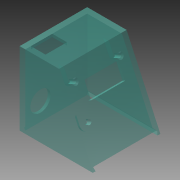
# Autodesk Inventor part: Caja temporizador
Saved by Autodesk Inventor 2014 (Build 180170000, 170)
## iProperties
Created: 2017-07-04
Part Number: Caja temporizador
Material: Generic
Document SubType Name: Modeling
Designer: resaj
Density: 1 g/cm^3
Appearance: Indoor Pool
Author: resaj
Autodesk Inventor part; units mm, degrees
ref_plane "YZ Plane" through (0, 0, 0) normal (1, 0, 0) x (0, 1, 0)
ref_plane "XZ Plane" through (0, 0, 0) normal (0, 1, 0) x (-1, 0, 0)
sketch "Sketch1" plane through (0, 0, 0) normal (0, 0, 1) x (1, 0, 0)
  line L0 (0, 0) -> (0, 65)
  line L1 (0, 65) -> (35, 65)
  line L2 (35, 65) -> (65, 0)
  line L3 (65, 0) -> (0, 0)
  line L4 (35, 65) -> (19.5647, 57.876) construction
  line L5 (19.5647, 57.876) -> (40.0985, 13.386) construction
  line L6 (40.0985, 13.386) -> (55.5339, 20.51) construction
  line L7 (5, 65) -> (5, 39) construction
  line L8 (5, 39) -> (17.8, 39) construction
  line L9 (17.8, 39) -> (17.8, 65) construction
  line L10 (0, 23.6) -> (40, 23.6) construction
  line L11 (40, 23.6) -> (40, 6) construction
  line L12 (40, 6) -> (0, 6) construction
  line L13 (0, 26.5) -> (11, 26.5) construction
  line L14 (11, 26.5) -> (11, 23.6) construction
  line L15 (11, 6) -> (11, 3.1) construction
  line L16 (11, 3.1) -> (0, 3.1) construction
  dimension "d27" = 17
  dimension "d28" = 12.8
  dimension "d29" = 5
  dimension "d31" = 40
  dimension "d32" = 17.6
  dimension "d33" = 26
  dimension "d34" = 35
  dimension "d35" = 65
  dimension "d36" = 23.4
  dimension "d37" = 11
  dimension "d38" = 49
  dimension "d39" = 65
  dimension "d40" = 6
  constraints: 34 end point, 12 perpendicular, 9 point on line, 2 equal length, 2 parallel, 1 collinear, 1 vertical
  measures "d27" distance of L1.end L4.end
  measures "d28" distance of L7.end L8.end
  measures "d29" distance between parallel lines of L0 L7
  measures "d31" distance of L10.start L10.end
  measures "d32" distance of L10.end L11.end
  measures "d33" distance of L7.start L7.end
  measures "d34" distance of L0.end L1.end
  measures "d35" distance of L2.end L0.start
  measures "d36" distance between parallel lines of L16 L13
  measures "d37" distance of L13.start L13.end
  measures "d38" distance of L4.end L5.end
  measures "d39" distance of L0.start L0.end
  measures "d40" distance between parallel lines of L3 L12
extrude "Extrusion1" add sketch "Sketch1" along normal blind 2.5
sketch "Sketch2" plane through (0, 0, 2.5) normal (0, 0, 1) x (1, 0, 0)
  line L0 (0, 65) -> (0, 0) projected
  line L1 (0, 0) -> (65, 0) projected
  line L2 (65, 0) -> (35, 65) projected
  line L3 (35, 65) -> (0, 65) projected
  line L4 (2.5, 2.5) -> (2.5, 62.5)
  line L5 (2.5, 62.5) -> (33.4004, 62.5)
  line L6 (33.4004, 62.5) -> (61.0927, 2.5)
  line L7 (61.0927, 2.5) -> (2.5, 2.5)
  line L8 (2.5, 2.5) -> (2.5, 0)
  line L9 (60.862, 3) -> (63.6154, 3)
  dimension "d2" = 2.5
  dimension "d3" = 3
  constraints: 12 end point, 3 point on line, 2 perpendicular, 3 other
  measures "d2" distance between parallel lines of L0 L4
  measures "d3" distance between parallel lines of L1 L9
extrude "Extrusion2" add sketch "Sketch2" along normal blind 55 contours L3 L2 L9 L6 L5 L4 L8 L1 L0
sketch "Sketch3" plane through (0, 0, 57.5) normal (0, 0, 1) x (1, 0, 0)
  line L0 (0, 65) -> (0, 0) projected
  line L1 (0, 0) -> (2.5, 0) projected
  line L2 (2.5, 0) -> (2.5, 62.5) projected
  line L3 (2.5, 62.5) -> (33.4004, 62.5) projected
  line L4 (33.4004, 62.5) -> (60.862, 3) projected
  line L5 (60.862, 3) -> (63.6154, 3) projected
  line L6 (63.6154, 3) -> (35, 65) projected
  line L7 (35, 65) -> (0, 65) projected
  line L8 (63.6154, 3) -> (65, 0)
  line L9 (65, 0) -> (2.5, 0)
  constraints: 4 end point, 1 collinear, 1 horizontal
extrude "Extrusion3" add sketch "Sketch3" along normal blind 2.5
sketch "Sketch4" plane through (0, 65, 0) normal (0, 1, 0) x (1, 0, 0)
  line L0 (5, -36) -> (18, -36)
  line L1 (18, -36) -> (18, -55)
  line L2 (18, -55) -> (5, -55)
  line L3 (5, -55) -> (5, -36)
  line L4 (0, 0) -> (0, -60) projected
  line L5 (35, -60) -> (0, -60) projected
  line L6 (4.1, -35.1) -> (18.9, -35.1) construction
  line L7 (18.9, -35.1) -> (18.9, -55.9) construction
  line L8 (18.9, -55.9) -> (4.1, -55.9) construction
  line L9 (4.1, -55.9) -> (4.1, -35.1) construction
  line L10 (5, -45.5) -> (4.1, -45.5) construction
  line L11 (18, -45.5) -> (18.9, -45.5) construction
  line L12 (11.5, -36) -> (11.5, -35.1) construction
  line L13 (11.5, -55) -> (11.5, -55.9) construction
  dimension "d41" = 13
  dimension "d42" = 19
  dimension "d43" = 14.8
  dimension "d44" = 20.8
  dimension "d45" = 5
  dimension "d46" = 5
  constraints: 24 end point, 8 midpoint, 4 parallel, 3 horizontal, 2 perpendicular, 1 vertical
  measures "d41" distance of L0.start L0.end
  measures "d42" distance of L0.end L1.end
  measures "d43" distance of L7.end L8.end
  measures "d44" distance of L8.end L6.start
  measures "d45" distance between parallel lines of L4 L3
  measures "d46" distance between parallel lines of L2 L5
extrude "Extrusion4" cut sketch "Sketch4" against normal through all
sketch "Sketch5" plane through (35, 65, 60) normal (0.9079594, 0.4190582, 0) x (0, 0, -1)
  line L0 (16.32, -14.8) -> (46.52, -14.8)
  line L1 (46.52, -14.8) -> (46.52, -29)
  line L2 (46.52, -29) -> (16.32, -29)
  line L3 (16.32, -29) -> (16.32, -14.8)
  circle A0 centre (9.42, -40.9) radius 1.95
  line L4 (60, -71.5891) -> (57.5, -71.5891) projected
  circle A1 centre (49.02, -12.9) radius 1.6
  circle A2 centre (9.02, -12.9) radius 1.6
  line L5 (9.02, -12.9) -> (49.02, -12.9) construction
  line L6 (60, 0) -> (0, 0) projected
  line L7 (3.5, -10) -> (53.82, -10) construction
  line L8 (53.82, -10) -> (53.82, -59.3) construction
  line L9 (53.82, -59.3) -> (3.5, -59.3) construction
  line L10 (3.5, -59.3) -> (3.5, -10) construction
  line L11 (0, -71.5891) -> (0, 0) projected
  point P0 (60, -44.3503)
  dimension "d17" = 40
  dimension "d18" = 3.2
  dimension "d19" = 30.2
  dimension "d20" = 14.2
  dimension "d47" = 2.5
  dimension "d48" = 1.9
  dimension "d49" = 28
  dimension "d50" = 39.6
  dimension "d51" = 50.32
  dimension "d52" = 4.8
  dimension "d53" = 49.3
  dimension "d54" = 2.9
  dimension "d55" = 10
  dimension "d72" = 3.5
  dimension "d73" = 3.9
  constraints: 18 end point, 5 parallel, 3 centre point, 2 horizontal, 2 perpendicular, 1 equal radius
  measures "d17" distance of L5.start L5.end
  measures "d18" diameter of A1
  measures "d19" distance of L1.end L2.end
  measures "d20" distance of L0.end L1.end
  measures "d47" distance from line of L1 L5.end
  measures "d48" vertical distance of L0.end L5.end
  measures "d49" vertical distance of A0.centre L5.start
  measures "d50" horizontal distance of A0.centre L5.end
  measures "d51" distance of L7.start L7.end
  measures "d52" distance from line of L8 L5.end
  measures "d53" distance of L7.end L8.end
  measures "d54" distance from line of L7 L5.start
  measures "d55" distance between parallel lines of L7 L6
  measures "d72" distance between parallel lines of L11 L10
  measures "d73" diameter of A0
extrude "Extrusion5" cut sketch "Sketch5" against normal up to next
sketch "Sketch6" plane through (0, 0, 0) normal (-1, 0, 0) x (0, 0, 1)
  circle A0 centre (44, 16) radius 9
  line L0 (0, 0) -> (60, 0) projected
  line L1 (60, 65) -> (60, 0) projected
  dimension "d56" = 18
  dimension "d57" = 7
  dimension "d58" = 7
  constraints: 1 centre point
  measures "d56" diameter of A0
  measures "d57" distance edge to line of A0 L0
  measures "d58" distance edge to line of A0 L1
extrude "Extrusion6" cut sketch "Sketch6" against normal up to next
ref_plane "Work Plane1" through (65, 0, 57.5) normal (1, 0, 0) x (0, 0, -1)
sketch "Sketch7" plane through (65, 0, 57.5) normal (1, 0, 0) x (0, 0, -1)
  line L0 (57.5, 65) -> (57.5, 0) projected
  line L1 (57.5, 65) -> (-2.5, 65) projected
  line L2 (-2.5, 0) -> (-2.5, 65) projected
  line L3 (0, 0) -> (-2.5, 0) projected
  line L4 (0, 0) -> (0, 3) projected
  line L5 (55, 3) -> (0, 3) projected
  line L6 (55, 0) -> (55, 3) projected
  line L7 (57.5, 0) -> (55, 0) projected
  line L8 (13.82, 38.6692) -> (13.82, 51.5622) projected
  line L9 (13.82, 51.5622) -> (44.02, 51.5622) projected
  line L10 (44.02, 51.5622) -> (44.02, 38.6692) projected
  line L11 (44.02, 38.6692) -> (13.82, 38.6692) projected
  ellipse E0 centre (6.92, 27.8645) end of major axis (4.97, 27.8645) minor radius 1.7705 projected
  line L12 (0, 0) -> (-1, 3)
  line L13 (-1, 3) -> (0, 3)
  line L14 (55, 3) -> (56, 3)
  line L15 (56, 3) -> (55, 0)
  dimension "d59" = 1
  constraints: 8 end point, 2 collinear, 1 horizontal, 1 other
  measures "d59" distance of L12.end L4.end
extrude "Extrusion7" cut sketch "Sketch7" against normal up to surface (62.5 mm away) contours L6 L14 L15 | L12 L13 L4
fillet "Fillet1" radius 0.5 2 edges at (33.0577, 3, 58.5) (33.0577, 3, 1.5)
sketch "Sketch8" plane through (60.862, 3, 2.5) normal (-0.9079594, -0.4190582, 0) x (0, 0, 1)
  circle A0 centre (8.48, 54.2311) radius 1.6 projected
  circle A1 centre (48.48, 54.2311) radius 1.6 projected
  arc A2 (45.48, 54.2311) -> (51.48, 54.2311) centre (48.48, 54.2311) ccw
  line L0 (10.98, 52.3311) -> (41.18, 52.3311) projected
  line L1 (5.48, 54.2311) -> (5.48, 58.2311)
  line L2 (11.48, 58.2311) -> (11.48, 54.2311)
  line L3 (45.48, 54.2311) -> (45.48, 58.2311)
  line L4 (51.48, 58.2311) -> (51.48, 54.2311)
  line L5 (0, 65.5316) -> (55, 65.5316) projected
  arc A3 (5.48, 54.2311) -> (11.48, 54.2311) centre (8.48, 54.2311) ccw
  line L6 (5.48, 58.2311) -> (11.48, 58.2311)
  line L7 (45.48, 58.2311) -> (51.48, 58.2311)
  point P0 (-2.5, 22.7808)
  point P1 (6.9, 65.5316)
  point P2 (12.9, 65.5316)
  point P3 (46.9, 65.5316)
  point P4 (52.9, 65.5316)
  dimension "d60" = 3
  dimension "d61" = 4
  constraints: 12 end point, 6 perpendicular, 4 point on circle, 4 point on line, 4 tangent, 3 parallel, 2 centre point, 2 coincident, 1 equal radius
  measures "d60" radius of A3
  measures "d61" distance of L2.start L2.end
extrude "Extrusion8" add sketch "Sketch8" along normal blind 4.8
sketch "Sketch12" plane through (36.4597, 55.8715, 53.98) normal (-0.4190582, 0.9079594, 0) x (0.9079594, 0.4190582, 0)
  line L0 (0, 6) -> (0, 0) projected
  line L1 (0, 6) -> (-4.8, 6) projected
  line L2 (-4.8, 0) -> (-4.8, 6) projected
  line L3 (0, 0) -> (-4.8, 0) projected
  line L4 (0, 46) -> (0, 40) projected
  line L5 (0, 46) -> (-4.8, 46) projected
  line L6 (-4.8, 40) -> (-4.8, 46) projected
  line L7 (0, 40) -> (-4.8, 40) projected
  point P0 (-56.5174, 53.98)
extrude "Extrusion11" add sketch "Sketch12" along normal up to next
sketch "Sketch13" plane through (35, 65, 60) normal (0.9079594, 0.4190582, 0) x (0, 0, -1)
  circle A0 centre (49.02, -12.9) radius 1.6 projected
  circle A1 centre (9.02, -12.9) radius 1.6 projected
  point P0 (60, -44.3503)
hole "Hole1" at (40.4059, 53.2873, 50.98) at (40.4059, 53.2873, 10.98) direction (-0.9079594, -0.4190582, 0) diameter 3 depth 20 tip angle 118 countersink diameter 5.5 countersink angle 90
sketch "Sketch14" plane through (60.862, 3, 2.5) normal (-0.9079594, -0.4190582, 0) x (0, 0, 1)
  line L0 (55, 65.5316) -> (55, 0) projected
  line L1 (10.98, 52.3311) -> (41.18, 52.3311) projected
  circle A0 centre (48.08, 26.2311) radius 1.95 projected
  arc A1 (42.08, 26.2311) -> (54.08, 26.2311) centre (48.08, 26.2311) ccw
  line L2 (42.08, 26.2311) -> (42.08, 33.9811)
  line L3 (42.08, 33.9811) -> (54.08, 33.9811)
  line L4 (54.08, 33.9811) -> (54.08, 26.2311)
  arc A2 (54.08, 26.2311) -> (42.08, 26.2311) centre (48.08, 26.2311) ccw construction
  point P0 (-2.5, 22.7808)
  dimension "d71" = 12
  dimension "d80" = 1.75
  constraints: 6 end point, 4 point on circle, 3 tangent, 2 centre point, 2 perpendicular, 1 coincident, 1 parallel
  measures "d71" diameter of A1
  measures "d80" distance edge to line of A2 L3
extrude "Extrusion12" add sketch "Sketch14" along normal blind 1.75
chamfer "Chamfer1" distance 1.75 angle 45 1 edges at (45.033, 33.1201, 50.58)
body "Solid1"
